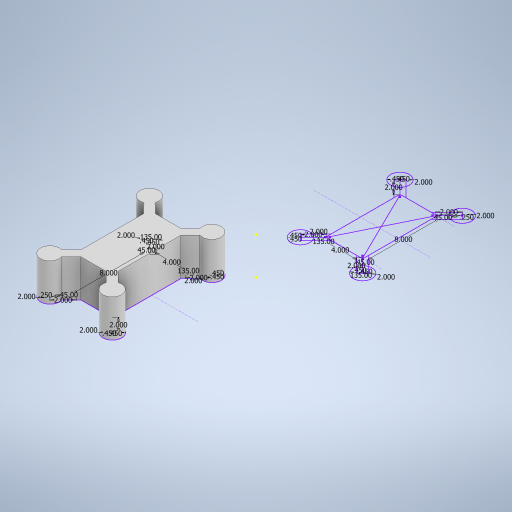
# Autodesk Inventor part: Part1
Saved by Autodesk Inventor 2023.2 (Build 272271030, 271C)
## iProperties
Created: 2023-03-18
Part Number: Part1
Material: Generic
Document SubType Name: Modeling
Designer: vinay
Density: 1 g/cm^3
Appearance: Default
Author: vinay
Autodesk Inventor part; units mm, degrees
ref_plane "YZ Plane" through (0, 0, 0) normal (1, 0, 0) x (0, 1, 0)
ref_plane "XZ Plane" through (0, 0, 0) normal (0, 1, 0) x (-1, 0, 0)
ref_plane "XY Plane" through (0, 0, 0) normal (0, 0, 1) x (1, 0, 0)
sketch "Sketch1" plane through (0, 0, 0) normal (0, 1, 0) x (-1, 0, 0)
  line L0 (106.9403, 291.2572) -> (195.8403, 291.2572)
  line L1 (202.1903, 284.9072) -> (202.1903, 94.4072)
  line L2 (195.8403, 88.0572) -> (106.9403, 88.0572)
  line L3 (100.5903, 94.4072) -> (100.5903, 284.9072)
  arc A0 (202.1903, 284.9072) -> (195.8403, 291.2572) centre (195.8403, 284.9072) ccw
  arc A1 (195.8403, 88.0572) -> (202.1903, 94.4072) centre (195.8403, 94.4072) ccw
  arc A2 (106.9403, 291.2572) -> (100.5903, 284.9072) centre (106.9403, 284.9072) ccw
  arc A3 (100.5903, 94.4072) -> (106.9403, 88.0572) centre (106.9403, 94.4072) ccw
  line L4 (200.3304, 289.3973) -> (236.2514, 325.3183)
  line L5 (200.3304, 289.3973) -> (251.1304, 289.3973) construction
  line L6 (200.3304, 89.917) -> (236.2514, 53.996)
  line L7 (200.3304, 89.917) -> (251.1304, 89.917) construction
  line L8 (102.4502, 289.3973) -> (66.5291, 325.3183) construction
  line L9 (102.4502, 89.917) -> (66.5291, 53.996)
  line L10 (102.4502, 89.917) -> (153.2502, 89.917) construction
  arc A4 (228.2944, 301.1968) -> (212.13, 317.3613) centre (236.2514, 325.3183) ccw
  circle A5 centre (236.2514, 53.996) radius 25.4
  arc A6 (90.6506, 317.3613) -> (74.4862, 301.1968) centre (66.5291, 325.3183) ccw
  circle A7 centre (66.5291, 53.996) radius 25.4
  line L11 (66.5291, 325.3183) -> (58.4469, 317.2361)
  line L12 (58.4469, 317.2361) -> (100.5903, 275.0927)
  line L13 (66.5291, 325.3183) -> (74.6114, 333.4006)
  line L14 (74.6114, 333.4006) -> (116.7547, 291.2572)
  line L15 (236.2514, 325.3183) -> (228.1692, 333.4006)
  line L16 (228.1692, 333.4006) -> (236.2514, 325.3183)
  line L17 (236.2514, 325.3183) -> (244.3337, 317.2361)
  line L18 (228.1692, 333.4006) -> (186.0258, 291.2572)
  line L19 (244.3337, 317.2361) -> (202.1903, 275.0927)
  line L20 (293.8482, 183.4348) -> (-26.9886, 183.4348) construction
  line L21 (236.2514, 53.996) -> (228.1692, 45.9138)
  line L22 (236.2514, 53.996) -> (247.6814, 53.996) construction
  line L23 (236.2514, 53.996) -> (244.3337, 62.0783)
  line L24 (228.1692, 45.9138) -> (186.0258, 88.0572)
  line L25 (244.3337, 62.0783) -> (202.1903, 104.2216)
  line L26 (66.5291, 53.996) -> (74.6114, 45.9138)
  line L27 (66.5291, 53.996) -> (58.4469, 62.0783)
  line L28 (58.4469, 62.0783) -> (100.5903, 104.2216)
  line L29 (74.6114, 45.9138) -> (116.7547, 88.0572)
  circle A8 centre (66.5291, 325.3183) radius 25.4
  circle A9 centre (236.2514, 325.3183) radius 25.4
  line L30 (66.5291, 325.3183) -> (102.4502, 289.3973)
  point P0 (0, 0)
  point P1 (202.1903, 88.0572)
  point P2 (202.1903, 291.2572)
  point P3 (100.5903, 88.0572)
  point P4 (228.2944, 78.1175)
  point P5 (212.13, 61.953)
  point P6 (74.4862, 78.1175)
  point P7 (90.6506, 61.953)
  point P8 (74.4862, 301.1968)
  dimension "d0" = 101.6
  dimension "d1" = 203.2
  dimension "d2" = 6.35
  dimension "d3" = 50.8
  dimension "d4" = 45
  dimension "d5" = 50.8
  dimension "d6" = 45
  dimension "d7" = 50.8
  dimension "d8" = 50.8
  dimension "d9" = 135
  dimension "d10" = 50.8
  dimension "d11" = 50.8
  dimension "d12" = 50.8
  dimension "d13" = 50.8
  dimension "d14" = 11.43
  dimension "d15" = 11.43
  dimension "d16" = 11.43
  dimension "d17" = 135
  dimension "d18" = 11.43
  dimension "d19" = 11.43
  dimension "d20" = 11.43
  constraints: 62 end point, 24 point on line, 16 point on circle, 10 centre point, 10 equal length, 8 perpendicular, 8 tangent, 6 horizontal, 5 equal radius, 4 coincident
  measures "d0" distance of point (202.19, 88.057) point (100.59, 88.057)
  measures "d1" distance of point (202.19, 291.257) point (202.19, 88.057)
  measures "d2" radius of A0
  measures "d3" distance of L4.start L4.end
  measures "d4" angle of L5 L4
  measures "d5" distance of L6.start L6.end
  measures "d6" angle of L6 L7
  measures "d7" distance of L8.start L8.end
  measures "d8" distance of L9.start L9.end
  measures "d9" angle of L9 L10
  measures "d10" diameter of A4
  measures "d11" diameter of A5
  measures "d12" diameter of A6
  measures "d13" diameter of A7
  measures "d14" distance of L11.start L11.end
  measures "d15" distance of L13.start L13.end
  measures "d16" distance of L21.start L21.end
  measures "d17" angle of L21 L22
  measures "d18" distance of L21.start L23.end
  measures "d19" distance of L26.start L26.end
  measures "d20" distance of L26.start L27.end
extrude "Extrusion1" add sketch "Sketch1" along normal blind 101.6 contours L0 A0 L1 A1 L2 A3 L3 A2
extrude "Extrusion2" add sketch "Sketch1" along normal blind 101.6 contours A2 L30 A8 L14 L0 | A2 L3 L12 A8 L30 | L18 A9 L4 A0 L0 | L14 L13 L11 L12 A6 | A8 L30 L13 L14 | A8 L12 L11 L30 | A4 L19 L17 L15 L18 | L18 L15 L4 A9 | L4 A9 L19 L1 A0 | L4 L17 L19 A9 | L3 A3 L9 A7 L28 | L28 L27 L26 L29 A7 | A7 L9 L27 L28 | A3 L2 L29 A7 L9 | A7 L29 L26 L9 | L25 A5 L6 A1 L1 | L25 L23 L6 A5 | A5 L24 L21 L23 L25 | L6 A5 L24 L2 A1 | L6 L21 L24 A5
extrude "Extrusion3" cut sketch "Sketch1" along normal blind 38.1 contours A2 L30 A8 L14 L0 | A2 L3 L12 A8 L30
sketch "Sketch2" plane through (0, 101.6, 0) normal (0, 1, 0) x (1, 0, 0)
  line L0 (106.9403, 291.2572) -> (195.8403, 291.2572)
  line L1 (202.1903, 284.9072) -> (202.1903, 94.4072)
  line L2 (195.8403, 88.0572) -> (106.9403, 88.0572)
  line L3 (100.5903, 94.4072) -> (100.5903, 284.9072)
  arc A0 (202.1903, 284.9072) -> (195.8403, 291.2572) centre (195.8403, 284.9072) ccw
  arc A1 (195.8403, 88.0572) -> (202.1903, 94.4072) centre (195.8403, 94.4072) ccw
  arc A2 (106.9403, 291.2572) -> (100.5903, 284.9072) centre (106.9403, 284.9072) ccw
  arc A3 (100.5903, 94.4072) -> (106.9403, 88.0572) centre (106.9403, 94.4072) ccw
  line L4 (200.3304, 289.3973) -> (236.2514, 325.3183)
  line L5 (200.3304, 289.3973) -> (251.1304, 289.3973) construction
  line L6 (200.3304, 89.917) -> (236.2514, 53.996)
  line L7 (200.3304, 89.917) -> (251.1304, 89.917) construction
  line L8 (102.4502, 289.3973) -> (66.5291, 325.3183) construction
  line L9 (102.4502, 89.917) -> (66.5291, 53.996)
  line L10 (102.4502, 89.917) -> (153.2502, 89.917) construction
  arc A4 (228.2944, 301.1968) -> (212.13, 317.3613) centre (236.2514, 325.3183) ccw
  circle A5 centre (236.2514, 53.996) radius 25.4
  arc A6 (90.6506, 317.3613) -> (74.4862, 301.1968) centre (66.5291, 325.3183) ccw
  circle A7 centre (66.5291, 53.996) radius 25.4
  line L11 (66.5291, 325.3183) -> (58.4469, 317.2361)
  line L12 (58.4469, 317.2361) -> (100.5903, 275.0927)
  line L13 (66.5291, 325.3183) -> (74.6114, 333.4006)
  line L14 (74.6114, 333.4006) -> (116.7547, 291.2572)
  line L15 (236.2514, 325.3183) -> (228.1692, 333.4006)
  line L16 (228.1692, 333.4006) -> (236.2514, 325.3183)
  line L17 (236.2514, 325.3183) -> (244.3337, 317.2361)
  line L18 (228.1692, 333.4006) -> (186.0258, 291.2572)
  line L19 (244.3337, 317.2361) -> (202.1903, 275.0927)
  line L20 (293.8482, 183.4348) -> (-26.9886, 183.4348) construction
  line L21 (236.2514, 53.996) -> (228.1692, 45.9138)
  line L22 (236.2514, 53.996) -> (247.6814, 53.996) construction
  line L23 (236.2514, 53.996) -> (244.3337, 62.0783)
  line L24 (228.1692, 45.9138) -> (186.0258, 88.0572)
  line L25 (244.3337, 62.0783) -> (202.1903, 104.2216)
  line L26 (66.5291, 53.996) -> (74.6114, 45.9138)
  line L27 (66.5291, 53.996) -> (58.4469, 62.0783)
  line L28 (58.4469, 62.0783) -> (100.5903, 104.2216)
  line L29 (74.6114, 45.9138) -> (116.7547, 88.0572)
  circle A8 centre (66.5291, 325.3183) radius 25.4
  circle A9 centre (236.2514, 325.3183) radius 25.4
  line L30 (66.5291, 325.3183) -> (102.4502, 289.3973)
  line L31 (200.3304, 289.3973) -> (102.4502, 89.917)
  line L32 (200.3304, 89.917) -> (102.4502, 289.3973)
  point P0 (0, 0)
  point P1 (202.1903, 88.0572)
  point P2 (202.1903, 291.2572)
  point P3 (100.5903, 88.0572)
  point P4 (228.2944, 78.1175)
  point P5 (212.13, 61.953)
  point P6 (74.4862, 78.1175)
  point P7 (90.6506, 61.953)
  point P8 (74.4862, 301.1968)
  dimension "d27" = 101.6
  dimension "d28" = 203.2
  dimension "d29" = 6.35
  dimension "d30" = 50.8
  dimension "d31" = 45
  dimension "d32" = 50.8
  dimension "d33" = 45
  dimension "d34" = 50.8
  dimension "d35" = 50.8
  dimension "d36" = 135
  dimension "d37" = 50.8
  dimension "d38" = 50.8
  dimension "d39" = 50.8
  dimension "d40" = 50.8
  dimension "d41" = 11.43
  dimension "d42" = 11.43
  dimension "d43" = 11.43
  dimension "d44" = 135
  dimension "d45" = 11.43
  dimension "d46" = 11.43
  dimension "d47" = 11.43
  constraints: 66 end point, 24 point on line, 16 point on circle, 10 centre point, 10 equal length, 8 perpendicular, 8 tangent, 6 horizontal, 5 equal radius, 4 coincident
  measures "d27" distance of point (202.19, 88.057) point (100.59, 88.057)
  measures "d28" distance of point (202.19, 291.257) point (202.19, 88.057)
  measures "d29" radius of A0
  measures "d30" distance of L4.start L4.end
  measures "d31" angle of L5 L4
  measures "d32" distance of L6.start L6.end
  measures "d33" angle of L6 L7
  measures "d34" distance of L8.start L8.end
  measures "d35" distance of L9.start L9.end
  measures "d36" angle of L9 L10
  measures "d37" diameter of A4
  measures "d38" diameter of A5
  measures "d39" diameter of A6
  measures "d40" diameter of A7
  measures "d41" distance of L11.start L11.end
  measures "d42" distance of L13.start L13.end
  measures "d43" distance of L21.start L21.end
  measures "d44" angle of L21 L22
  measures "d45" distance of L21.start L23.end
  measures "d46" distance of L26.start L26.end
  measures "d47" distance of L26.start L27.end
body "Solid1"
